y_pulley_holder_back (Autodesk Fusion 360 design; units mm, degrees)
Autodesk Fusion 360 part; units mm, degrees
sketch "Sketch1" plane through (0, 0, 0) normal (0, 1, 0) x (1, 0, 0)
  line L0 (0, 0) -> (11, 0)
  line L1 (11, 0) -> (11, -30)
  line L2 (11, -30) -> (0, -30)
  line L3 (0, -30) -> (0, 0)
  circle A0 centre (5.5, -15) radius 1.6
  circle A1 centre (5.5, -23) radius 2.5
  dimension "d1" = 30
  dimension "d2" = 11
  dimension "d3" = 3.2
  dimension "d4" = 5
  dimension "d5" = 15
  dimension "d6" = 8
  dimension "d7" = 5.5
  constraint horizontal L0
  constraint vertical L1
  constraint horizontal L2
  constraint vertical L3
  constraint coincident L0.start L3.end
  constraint vertical A0.centre A1.centre
  measures "d1" distance of L0.start L2.end
  measures "d2" distance of L1 L3
  measures "d3" diameter of A0
  measures "d4" diameter of A1
  measures "d5" distance of L0 A0.centre
  measures "d6" distance of A0.centre A1.centre
  measures "d7" distance of L3 A0.centre
extrude "Extrude1" add sketch "Sketch1" against normal blind 5 contours L0 L1 L2 L3 | A1
extrude "Extrude2" add sketch "Sketch1" against normal blind 2 from surface at -5 contours A1
fillet "Fillet1" radius 3 4 edges at (11, -2.5, 30) (0, -2.5, 30) (0, -2.5, 0) (11, -2.5, 0)
equation "d5 = d1 / 2"
equation "d7 = d2 / 2"
